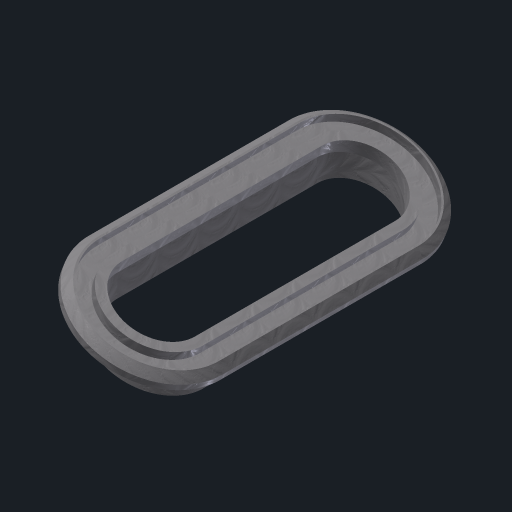
# Autodesk Inventor part: COMPUERTA_PLASTICO
Saved by Autodesk Inventor 2024.3 (Build 283343000, 343)
## iProperties
Created: 2024-07-04
Part Number: COMPUERTA_PLASTICO
Material: Steel, Mild, Welded
Document SubType Name: Modeling
Designer: Niler
Density: 7.85 g/cm^3
Appearance: Weld - Steel Mild
Author: Niler
Autodesk Inventor part; units mm, degrees
ref_plane "YZ Plane" through (0, 0, 0) normal (1, 0, 0) x (0, 1, 0)
ref_plane "XZ Plane" through (0, 0, 0) normal (0, 1, 0) x (-1, 0, 0)
ref_plane "XY Plane" through (0, 0, 0) normal (0, 0, 1) x (1, 0, 0)
sketch "Sketch1" plane through (0, 0, 0) normal (0, 1, 0) x (-1, 0, 0)
  line L0 (-101.5312, 175) -> (101.5312, 175)
  line L1 (101.5312, 175) -> (101.5312, -175)
  line L2 (101.5312, -175) -> (-101.5312, -175)
  line L3 (-101.5312, -175) -> (-101.5312, 175)
  line L4 (-101.5312, 175) -> (101.5312, -175) construction
  line L5 (101.5312, 175) -> (-101.5312, -175) construction
  point P0 (0, 0)
  dimension "d2" = 350
  constraints: 12 end point, 2 midpoint, 2 parallel, 1 horizontal, 1 perpendicular
  measures "d2" distance of L0.end L1.end
extrude "Extrusion1" add sketch "Sketch1" against normal blind 150
sketch "Sketch3" plane through (-101.5312, 0, 175) normal (0, 0, 1) x (-1, 0, 0)
  line L0 (0, 0) -> (-203.0624, 0) projected
  line L1 (-203.0624, 0) -> (-203.0624, 150) projected
  line L2 (-203.0624, 150) -> (0, 150) projected
  line L3 (0, 0) -> (0, 150) projected
  line L4 (0, 150) -> (-48.8156, 150)
  line L5 (0, 0) -> (47.3608, 0)
  line L6 (0, 0) -> (-203.0624, 81.2192)
  point P0 (-101.5312, 0)
  dimension "d7" = 158.2
  constraints: 6 end point, 2 horizontal, 1 point on line
  measures "d7" angle of L5 L6
extrude "Extrusion2" cut sketch "Sketch3" against normal through all contours L0 L1 L6
sketch "Sketch5" plane through (-101.5312, -150, 175) normal (0, 0, 1) x (1, 0, 0)
  line L0 (203.0624, 68.7808) -> (0, 150) projected
  line L1 (203.0624, 44.0093) -> (0, 125.2285)
  line L2 (0, 150) -> (0, 125.2285)
  line L3 (0, 150) -> (0, 0) projected
  line L4 (203.0624, 68.7808) -> (203.0624, 44.0093)
  line L5 (203.0624, 68.7808) -> (203.0624, 0) projected
  line L6 (203.0624, 0) -> (0, 0) projected
  point P0 (101.5312, 150)
  dimension "d13" = 23
  constraints: 8 end point, 1 parallel, 1 point on line, 1 vertical
  measures "d13" distance between parallel lines of L0 L1
extrude "Extrusion4" cut sketch "Sketch5" against normal through all contours L5 L6 L3 L1
sketch "Sketch4" plane through (0, 0, 0) normal (0, 1, 0) x (-1, 0, 0)
  line L0 (0, 110) -> (0, -110) construction
  line L1 (-55, 110) -> (-55, -110)
  line L2 (55, -110) -> (55, 110)
  arc A0 (55, 110) -> (-55, 110) centre (0, 110) ccw
  arc A1 (-55, -110) -> (55, -110) centre (0, -110) ccw
  line L3 (101.5312, -175) -> (-101.5312, -175) projected
  line L4 (101.5312, -175) -> (101.5312, 175) projected
  line L5 (-101.5312, 175) -> (101.5312, 175) projected
  line L6 (-101.5312, -175) -> (-101.5312, 175) projected
  line L7 (40, -110) -> (40, 110)
  arc A2 (40, 110) -> (-40, 110) centre (0, 110) ccw
  line L8 (-40, 110) -> (-40, -110)
  arc A3 (-40, -110) -> (40, -110) centre (0, -110) ccw
  point P0 (0, 0)
  dimension "d9" = 220
  dimension "d10" = 110
  dimension "d16" = 80
  constraints: 12 end point, 8 point on circle, 4 centre point, 4 tangent, 2 parallel, 1 midpoint, 1 vertical, 3 other
  measures "d9" distance of L0.start L0.end
  measures "d10" distance between parallel lines of L1 L2
  measures "d16" distance between parallel lines of L8 L7
extrude "Extrusion3" cut sketch "Sketch4" against normal through all
sketch "Sketch6" plane through (-55, -18.6111, 110) normal (0.3713678, 0.9284858, 0) x (0.9284858, -0.3713678, 0)
  line L0 (0, 220) -> (0, 0) projected
  ellipse E0 centre (59.2362, 0) end of major axis (118.4725, 0) minor radius 55 (0, 0) -> (118.4725, 0) ccw projected
  line L1 (118.4725, 0) -> (118.4725, 220) projected
  ellipse E1 centre (59.2362, 220) end of major axis (0, 220) minor radius 55 (118.4725, 220) -> (0, 220) ccw projected
  line L2 (102.3171, 220) -> (102.3171, 0) projected
  ellipse E2 centre (59.2362, 0) end of major axis (16.1553, 0) minor radius 40 (16.1553, 0) -> (102.3171, 0) ccw projected
  line L3 (16.1553, 0) -> (16.1553, 220) projected
  ellipse E3 centre (59.2362, 220) end of major axis (102.3171, 220) minor radius 40 (102.3171, 220) -> (16.1553, 220) ccw projected
  line L4 (-20, 0) -> (-20, 220)
  line L5 (138.4725, 220) -> (138.4725, 0)
  spline S0 degree 5 poles (-20, 220) (-20, 223.2067) (-19.8192, 226.4133) (-19.4575, 229.6064) (-17.1526, 243.1019) (-11.6689, 255.8711) (-5.7405, 264.7637) (8.9627, 280.1928) (27.8927, 290.0083) (38.1084, 293.3343) (59.2362, 296.6658) (80.364, 293.3343) (90.5798, 290.0083) (109.5097, 280.1928) (124.2129, 264.7637) (130.1413, 255.8711) (135.6251, 243.1019) (137.93, 229.6064) (138.2917, 226.4133) (138.4725, 223.2067) (138.4725, 220) knots 0 0 0 0 0 0 0.066163 0.066163 0.066163 0.282037 0.282037 0.282037 0.5 0.5 0.5 0.717963 0.717963 0.717963 0.933837 0.933837 0.933837 1 1 1 1 1 1
  spline S1 degree 5 poles (138.4725, 0) (138.4725, -3.2067) (138.2917, -6.4133) (137.93, -9.6064) (135.6251, -23.1019) (130.1413, -35.8711) (124.2129, -44.7637) (109.5097, -60.1928) (90.5798, -70.0083) (80.364, -73.3343) (59.2362, -76.6658) (38.1084, -73.3343) (27.8927, -70.0083) (8.9627, -60.1928) (-5.7405, -44.7637) (-11.6689, -35.8711) (-17.1526, -23.1019) (-19.4575, -9.6064) (-19.8192, -6.4133) (-20, -3.2067) (-20, 0) knots 0 0 0 0 0 0 0.066163 0.066163 0.066163 0.282037 0.282037 0.282037 0.5 0.5 0.5 0.717963 0.717963 0.717963 0.933837 0.933837 0.933837 1 1 1 1 1 1
  point P0 (44.1551, 110)
  dimension "d17" = 20
  constraints: 4 end point, 3 parallel, 2 horizontal alignment, 8 other
  measures "d17" distance between parallel lines of L0 L4
extrude "Extrusion5" add sketch "Sketch6" along normal blind 15 contours E1 L1 E0 L0 | L4 S0 L5 S1
sketch "Sketch7" plane through (-49.4295, -4.6839, 110) normal (0.3713678, 0.9284858, 0) x (0.9284858, -0.3713678, 0)
  line L0 (138.4725, 0) -> (138.4725, 220) projected
  spline S0 degree 5 poles (138.4725, 220) (138.4725, 223.2067) (138.2917, 226.4133) (137.93, 229.6064) (135.6251, 243.1019) (130.1413, 255.8711) (124.2129, 264.7637) (109.5097, 280.1928) (90.5798, 290.0083) (80.364, 293.3343) (59.2362, 296.6658) (38.1084, 293.3343) (27.8927, 290.0083) (8.9627, 280.1928) (-5.7405, 264.7637) (-11.6689, 255.8711) (-17.1526, 243.1019) (-19.4575, 229.6064) (-19.8192, 226.4133) (-20, 223.2067) (-20, 220) knots 0 0 0 0 0 0 0.066163 0.066163 0.066163 0.282037 0.282037 0.282037 0.5 0.5 0.5 0.717963 0.717963 0.717963 0.933837 0.933837 0.933837 1 1 1 1 1 1
  line L1 (-20, 220) -> (-20, 0) projected
  spline S1 degree 5 poles (-20, 0) (-20, -3.2067) (-19.8192, -6.4133) (-19.4575, -9.6064) (-17.1526, -23.1019) (-11.6689, -35.8711) (-5.7405, -44.7637) (8.9627, -60.1928) (27.8927, -70.0083) (38.1084, -73.3343) (59.2362, -76.6658) (80.364, -73.3343) (90.5798, -70.0083) (109.5097, -60.1928) (124.2129, -44.7637) (130.1413, -35.8711) (135.6251, -23.1019) (137.93, -9.6064) (138.2917, -6.4133) (138.4725, -3.2067) (138.4725, 0) knots 0 0 0 0 0 0 0.066163 0.066163 0.066163 0.282037 0.282037 0.282037 0.5 0.5 0.5 0.717963 0.717963 0.717963 0.933837 0.933837 0.933837 1 1 1 1 1 1
  line L2 (16.1553, 0) -> (16.1553, 220) projected
  ellipse E0 centre (59.2362, 220) end of major axis (16.1553, 220) minor radius 40 (102.3171, 220) -> (16.1553, 220) ccw projected
  line L3 (102.3171, 220) -> (102.3171, 0) projected
  ellipse E1 centre (59.2362, 0) end of major axis (102.3171, 0) minor radius 40 (16.1553, 0) -> (102.3171, 0) ccw projected
  line L4 (128.4725, 0) -> (128.4725, 220)
  line L5 (-10, 220) -> (-10, 0)
  line L6 (112.3171, 0) -> (112.3171, 220)
  line L7 (6.1553, 220) -> (6.1553, 0)
  spline S2 degree 5 poles (128.4725, 220.0001) (128.4723, 228.3573) (127.0436, 236.7168) (124.1803, 244.7436) (115.8689, 259.6179) (103.3089, 271.1427) (96.1383, 275.8932) (80.5639, 283.1417) (63.5597, 285.619) (54.9127, 285.619) (37.9085, 283.1417) (22.3342, 275.8932) (15.1636, 271.1427) (2.6035, 259.6179) (-5.7079, 244.7437) (-8.5711, 236.7168) (-9.9999, 228.3573) (-10, 220.0002) knots 0 0 0 0 0 0 0.198123 0.198123 0.198123 0.398885 0.398885 0.398885 0.601116 0.601116 0.601116 0.801878 0.801878 0.801878 1 1 1 1 1 1
  spline S3 degree 5 poles (-10, -0.0001) (-9.9999, -8.3573) (-8.5711, -16.7168) (-5.7079, -24.7436) (2.6035, -39.6179) (15.1636, -51.1427) (22.3342, -55.8932) (37.9086, -63.1417) (54.9127, -65.619) (63.5597, -65.619) (80.5639, -63.1417) (96.1383, -55.8932) (103.3089, -51.1427) (115.8689, -39.6179) (124.1803, -24.7436) (127.0436, -16.7168) (128.4723, -8.3573) (128.4725, -0.0001) knots 0 0 0 0 0 0 0.198123 0.198123 0.198123 0.398884 0.398884 0.398884 0.601116 0.601116 0.601116 0.801877 0.801877 0.801877 1 1 1 1 1 1
  spline S4 degree 5 poles (112.3171, 220) (112.3172, 222.1275) (112.1972, 224.2551) (111.9571, 226.3736) (110.4225, 235.3572) (106.7658, 243.8561) (102.8085, 249.7773) (92.9644, 260.0921) (80.2935, 266.6529) (73.4297, 268.883) (59.2362, 271.1171) (45.0427, 268.883) (38.179, 266.6529) (25.5081, 260.0921) (15.664, 249.7773) (11.7067, 243.8561) (8.0499, 235.3572) (6.5153, 226.3736) (6.2753, 224.2551) (6.1553, 222.1275) (6.1553, 220) knots 0 0 0 0 0 0 0.06568 0.06568 0.06568 0.280913 0.280913 0.280913 0.5 0.5 0.5 0.719087 0.719087 0.719087 0.93432 0.93432 0.93432 1 1 1 1 1 1
  spline S5 degree 5 poles (6.1553, 0) (6.1553, -2.1275) (6.2753, -4.2551) (6.5153, -6.3736) (8.0499, -15.3572) (11.7067, -23.8561) (15.664, -29.7773) (25.5081, -40.0921) (38.179, -46.6529) (45.0427, -48.883) (59.2362, -51.1171) (73.4297, -48.883) (80.2935, -46.6529) (92.9644, -40.0921) (102.8085, -29.7773) (106.7658, -23.8561) (110.4225, -15.3572) (111.9571, -6.3736) (112.1972, -4.2551) (112.3172, -2.1275) (112.3171, 0) knots 0 0 0 0 0 0 0.06568 0.06568 0.06568 0.280913 0.280913 0.280913 0.5 0.5 0.5 0.719087 0.719087 0.719087 0.93432 0.93432 0.93432 1 1 1 1 1 1
  point P0 (44.1551, 110)
  dimension "d20" = 10
  dimension "d21" = 10
  constraints: 8 end point, 6 horizontal alignment, 6 parallel, 10 other
extrude "Extrusion6" cut sketch "Sketch7" against normal blind 10 contours S3 L5 S2 L4
chamfer "Chamfer1" distance 8 angle 45 4 edges at (5.5705, -26.6823, 185.0001) (79.1402, -56.1081, 0) (5.5705, -26.6823, -185.0001) (-67.9992, 2.7435, 0)
body "Solid1"
